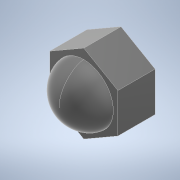
# Autodesk Inventor part: M3 Acorn Nut
Saved by Autodesk Inventor 2022 (Build 260153000, 153)
## iProperties
Created: 2022-05-12
Part Number: M3 Acorn Nut
Material: Generic
Document SubType Name: Modeling
Designer: Nick
Density: 1 g/cm^3
Appearance: Smooth - Black
Author: Nick
Autodesk Inventor part; units mm, degrees
ref_plane "YZ Plane" through (0, 0, 0) normal (1, 0, 0) x (0, 1, 0)
ref_plane "XZ Plane" through (0, 0, 0) normal (0, 1, 0) x (-1, 0, 0)
ref_plane "XY Plane" through (0, 0, 0) normal (0, 0, 1) x (1, 0, 0)
sketch "Sketch1" plane through (0, 0, 0) normal (0, 0, 1) x (1, 0, 0)
  line L0 (2.75, 1.5877) -> (2.75, -1.5877)
  line L1 (2.75, -1.5877) -> (0, -3.1754)
  line L2 (0, -3.1754) -> (-2.75, -1.5877)
  line L3 (-2.75, -1.5877) -> (-2.75, 1.5877)
  line L4 (-2.75, 1.5877) -> (0, 3.1754)
  line L5 (0, 3.1754) -> (2.75, 1.5877)
  circle A0 centre (0, 0) radius 1.5
  dimension "d0" = 5.5
  dimension "d1" = 3
  constraints: 12 end point, 2 coincident, 1 centre point, 1 vertical, 13 other
  measures "d0" distance between parallel lines of L3 L0
  measures "d1" diameter of A0
extrude "Extrusion1" add sketch "Sketch1" along normal blind 3
sketch "Sketch2" plane through (0, 0, 0) normal (1, 0, 0) x (0, 1, 0)
  line L0 (2.3816, 3) -> (2.3816, 4.1867) construction
  line L1 (2.3816, 4.1867) -> (0, 6.751) construction
  line L2 (0, 6.751) -> (-2.3816, 4.1867) construction
  line L3 (-2.3816, 4.1867) -> (-2.3816, 3) construction
  spline S0 degree 4 poles (2.3816, 3) (2.3816, 4.1867) (0, 6.751) (-2.3816, 4.1867) (-2.3816, 3) knots 1 1 1 1 1 2 2 2 2 2
  line L4 (0.553, 5) -> (-1.6263, 5)
  line L5 (-3.1754, 0) -> (-1.5877, 0) projected
  line L6 (-1.5877, 3) -> (1.5877, 3) projected
  line L7 (-3.1754, 3) -> (-1.5877, 3) projected
  line L8 (1.5877, 3) -> (3.1754, 3) projected
  line L9 (2.3816, 3) -> (-2.3816, 3)
  line L10 (0, 3) -> (0, 6.751)
  line L11 (1.5877, 3) -> (-1.5877, 3) projected
  point P0 (0, 0)
  point P1 (0, 5)
  dimension "d4" = 5
  constraints: 6 end point, 3 midpoint, 2 horizontal, 2 perpendicular, 2 vertical, 1 coincident, 1 horizontal alignment, 1 point on line, 1 vertical alignment, 3 other
  measures "d4" distance between parallel lines of L5 L4
revolve "Revolution1" add sketch "Sketch2" angle 360 about axis through (0, 0, 3) along (0, 0, 1) contours L8 L6 L10 S0
thread "Thread1" size "M3x0.5" class "6H" standard "ANSI Metric M Profile" full length
body "Solid1"
